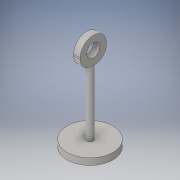
# Autodesk Inventor part: Pneumatickolben_Kolbenkreis
Saved by Autodesk Inventor 2016 (Build 200138000, 138)
## iProperties
Created: 2019-05-08
Part Number: Pneumatickolben_Kolbenkreis
Material: Generisch
Document SubType Name: Modeling
Designer: Teilnehmer
Density: 1 g/cm^3
Appearance: Vorgabe
Author: Teilnehmer
Autodesk Inventor part; units mm, degrees
ref_plane "YZ Plane" through (0, 0, 0) normal (1, 0, 0) x (0, 1, 0)
ref_plane "XZ Plane" through (0, 0, 0) normal (0, 1, 0) x (-1, 0, 0)
ref_plane "XY Plane" through (0, 0, 0) normal (0, 0, 1) x (1, 0, 0)
sketch "Skizze1" plane through (0, 0, 0) normal (0, 0, 1) x (1, 0, 0)
  circle A0 centre (0, 0) radius 3.5
  dimension "d0" = 7
  constraints: 1 centre point, 1 coincident
  measures "d0" diameter of A0
extrude "Extrusion1" add sketch "Skizze1" along normal blind 1
sketch "Skizze2" plane through (0, 0, 1) normal (0, 0, 1) x (1, 0, 0)
  circle A0 centre (0, 0) radius 0.5
  dimension "d3" = 1
  constraints: 1 centre point, 1 coincident
  measures "d3" diameter of A0
extrude "Extrusion2" add sketch "Skizze2" along normal blind 14
sketch "Skizze4" plane through (0, 0, 15) normal (0, 0, 1) x (1, 0, 0)
  line L0 (-0.5, -2) -> (0.5, -2)
  line L1 (0.5, -2) -> (0.5, 2)
  line L2 (0.5, 2) -> (-0.5, 2)
  line L3 (-0.5, 2) -> (-0.5, -2)
  circle A0 centre (0, 0) radius 0.5 projected
  dimension "d25" = 1
  dimension "d26" = 4
  dimension "d27" = 2
  constraints: 8 end point, 2 parallel, 1 horizontal, 1 perpendicular, 1 tangent
  measures "d25" distance of L1.end L2.end
  measures "d26" distance of L0.end L1.end
  measures "d27" distance from line of point (0, 0) L2
extrude "Extrusion4" add sketch "Skizze4" against normal blind 4 contours L3 A0 L1 L0 | L3 L2 L1 A0
sketch "Skizze6" plane through (-0.5, -2, 15) normal (-1, 0, 0) x (0, 0, 1)
  circle A0 centre (-2, 2) radius 1
  line L0 (0, 4) -> (-4, 4) projected
  line L1 (0, 4) -> (0, 0) projected
  point P0 (-15, 2)
  dimension "d31" = 2
  dimension "d32" = 2
  dimension "d33" = 2
  constraints: 1 centre point
  measures "d31" diameter of A0
  measures "d32" distance from line of L0 A0.centre
  measures "d33" distance from line of L1 A0.centre
extrude "Extrusion5" cut sketch "Skizze6" against normal blind 1
sketch "Skizze10" plane through (-0.5, -2, 15) normal (-1, 0, 0) x (0, 0, 1)
  point P0 (-15, 2)
fillet "Rundung9" radius 2 1 edges at (0, 2, 15)
fillet "Rundung10" radius 2 1 edges at (0, -2, 15)
fillet "Rundung11" radius 1.75 1 edges at (0, -2, 11)
fillet "Rundung12" radius 1.75 1 edges at (0, 2, 11)
